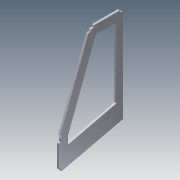
# Autodesk Inventor part: TopSidePanel-Left
Saved by Autodesk Inventor 2014 (Build 180170000, 170)
## iProperties
Created: 2014-08-11
Part Number: TopSidePanel-Left
Material: Generic
Document SubType Name: Modeling
Designer: Peele
Density: 1 g/cm^3
Appearance: White
Author: Peele
Autodesk Inventor part; units mm, degrees
ref_plane "YZ Plane" through (0, 0, 0) normal (1, 0, 0) x (0, 1, 0)
ref_plane "XZ Plane" through (0, 0, 0) normal (0, 1, 0) x (-1, 0, 0)
ref_plane "XY Plane" through (0, 0, 0) normal (0, 0, 1) x (1, 0, 0)
sketch "Sketch1" plane through (0, 0, 0) normal (1, 0, 0) x (0, 1, 0)
  line L0 (0, 325) -> (0, 0)
  line L1 (0, 0) -> (-186, 0)
  line L2 (-186, 0) -> (-186, 85)
  line L3 (-2.414491, 325) -> (0, 325)
  line L4 (0, 325) -> (-95, 325)
  line L5 (-95, 325) -> (-186, 85)
  dimension "d0" = 325
  dimension "d1" = 186
  dimension "d2" = 85
  dimension "d3" = 95
  dimension "d33" = 240
  dimension "d34" = 91
  constraints: 12 end point, 2 parallel, 1 collinear, 1 perpendicular, 1 vertical
  measures "d0" distance of L0.start L0.end
  measures "d1" distance of L0.end L1.end
  measures "d2" distance of L1.end L2.end
  measures "d3" distance of L0.start L4.end
  measures "d33" vertical distance of L2.end L4.end
  measures "d34" horizontal distance of L4.end L2.end
extrude "Extrusion1" add sketch "Sketch1" along normal blind 6
sketch "Sketch2" plane through (6, 0, 0) normal (1, 0, 0) x (0, 0, -1)
  line L0 (-325, 0) -> (-325, -95) projected
  line L1 (-325, -8.1) -> (-331, -8.1)
  line L2 (-331, -8.1) -> (-331, -86.9)
  line L3 (-331, -86.9) -> (-325, -86.9)
  line L4 (-325, -86.9) -> (-325, -8.1)
  line L5 (-85, -186) -> (0, -186) projected
  line L6 (0, -186) -> (0, 0) projected
  line L7 (-76.9, -186) -> (-8.1, -186)
  line L8 (-8.1, -186) -> (-8.1, -192)
  line L9 (-8.1, -192) -> (-76.9, -192)
  line L10 (-76.9, -192) -> (-76.9, -186)
  line L11 (-325, -95) -> (-331, -86.9) construction
  line L12 (-325, 0) -> (-331, -8.1) construction
  dimension "d6" = 6
  dimension "d12" = 6
  dimension "d13" = 8.1
  dimension "d47" = 8.1
  dimension "d48" = 8.1
  constraints: 20 end point, 4 parallel, 2 horizontal, 2 perpendicular, 2 point on line, 1 equal length
  measures "d6" distance of L1.start L1.end
  measures "d12" distance of L7.end L8.end
  measures "d13" distance between parallel lines of L8 L6
  measures "d47" distance from line of L0.end L3
  measures "d48" distance from line of L5.start L10
extrude "Extrusion2" add sketch "Sketch2" against normal blind 6
sketch "Sketch3" plane through (6, 0, 0) normal (1, 0, 0) x (0, 0, -1)
  line L0 (-317.426159, -97.871748) -> (-92.573841, -183.128252)
  line L1 (-92.573841, -183.128252) -> (-94.701061, -188.738504)
  line L2 (-94.701061, -188.738504) -> (-319.55338, -103.482)
  line L3 (-319.55338, -103.482) -> (-317.426159, -97.871748)
  line L4 (-325, -95) -> (-85, -186)
  dimension "d17" = 8.1
  dimension "d35" = 6
  dimension "d36" = 8.1
  constraints: 8 end point, 2 parallel, 1 collinear, 1 perpendicular
  measures "d17" distance from line of L4.start L3
  measures "d35" distance between parallel lines of L2 L0
  measures "d36" distance from line of L4.end L1
extrude "Extrusion3" add sketch "Sketch3" against normal blind 6
sketch "Sketch6" plane through (6, 0, 0) normal (1, 0, 0) x (0, 0, -1)
  line L0 (0, 0) -> (-325, 0) projected
  line L1 (0, -186) -> (0, 0) projected
  line L2 (0, -186) -> (-50, 25)
  line L3 (-50, 25) -> (0, 25)
  line L4 (0, 25) -> (0, -186)
  dimension "d38" = 50
  dimension "d39" = 25
  constraints: 6 end point, 2 perpendicular
  measures "d38" distance of L2.end L3.end
  measures "d39" distance between parallel lines of L3 L0
extrude "Extrusion6" cut sketch "Sketch6" against normal through all
fillet "Fillet2" radius 3 4 edges at (3, 0, 325) (3, -95, 325) (3, -186, 85) (3, -186, 0)
fillet "Fillet3" radius 2 6 edges at (3, -192, 8.1) (3, -192, 76.9) (3, -188.7385, 94.7011) (3, -103.482, 319.5534) (3, -86.9, 331) (3, -8.1, 331)
sketch "Sketch4" plane through (6, 0, 0) normal (1, 0, 0) x (0, 0, -1)
  line L0 (-323.06361, -95.734214) -> (-85.513953, -185.805126)
  line L1 (-323.06361, -95.734214) -> (-85.513953, -185.805126)
  line L2 (-44.075829, 0) -> (-322, 0)
  line L3 (-325, -3) -> (-325, -8.1)
  line L4 (-325, -8.1) -> (-329, -8.1)
  line L5 (-305, -20) -> (-305, -81.193921)
  line L6 (-305, -81.193921) -> (-84.450343, -164.819)
  line L7 (-84.450343, -164.819) -> (-84.450343, -20)
  line L8 (-84.450343, -20) -> (-305, -20)
  arc A0 (-85.513953, -185.805126) -> (-84.450343, -186) centre (-84.450343, -183) ccw
  line L9 (-8.1, -186) -> (-3.79398, -186)
  point P0 (-191.521346, -165.651434)
  point P1 (-106.085382, -201.605735)
  point P2 (-3, 0)
  point P3 (0, 0)
  dimension "d24" = 20
  dimension "d26" = 20
  dimension "d27" = 20
  constraints: 8 end point, 2 perpendicular, 1 parallel, 1 point on line, 3 other
  measures "d24" distance between parallel lines of L2 L8
  measures "d27" distance between parallel lines of L3 L5
extrude "Extrusion4" cut sketch "Sketch4" against normal through all
sketch "Sketch7" plane through (6, 0, 0) normal (1, 0, 0) x (0, 0, -1)
  line L0 (-84.450343, -20) -> (-84.450343, -164.819)
  line L1 (-0.874821, -182.308256) -> (-44.075829, 0)
  line L2 (-84.450343, -164.819) -> (-84.450343, -20)
  line L3 (-84.450343, -20) -> (-50.133044, -164.819)
  line L4 (-50.133044, -164.819) -> (-84.450343, -164.819)
  point P0 (0, 0)
  constraints: 6 end point, 1 collinear, 1 parallel, 1 perpendicular
extrude "Extrusion7" cut sketch "Sketch7" against normal through all
sketch "Sketch8" plane through (6, 0, 0) normal (1, 0, 0) x (0, 0, -1)
  line L0 (-84.450343, -20) -> (-50.133044, -164.819)
  line L1 (-50.133044, -164.819) -> (-84.450343, -164.819)
  line L2 (-305, -20) -> (-84.450343, -20)
  line L3 (-50.133044, -164.819) -> (-84.450343, -20)
  line L4 (-84.450343, -20) -> (-94.450343, -20)
  line L5 (-50.133044, -164.819) -> (-60.133044, -164.819)
  line L6 (-94.450343, -20) -> (-60.133044, -164.819)
  point P0 (0, 0)
  dimension "d44" = 10
  constraints: 8 end point, 2 equal length, 2 point on line
  measures "d44" distance of L5.end L0.end
extrude "Extrusion8" add sketch "Sketch8" against normal blind 6
fillet "Fillet4" radius 2 5 edges at (3, -164.819, 84.4503) (3, -164.819, 60.133) (3, -20, 94.4503) (3, -20, 305) (3, -81.1939, 305)
equation "\"d26\" = d24"
equation "\"d27\" = d24"
body "Solid1"
